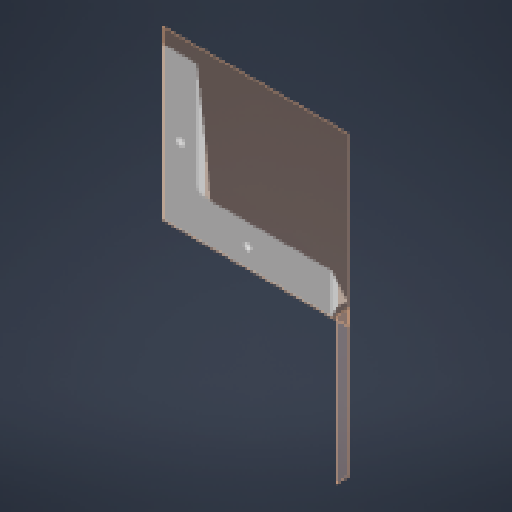
# Autodesk Inventor part: Base Gripper Support
Saved by Autodesk Inventor 2026.1 (Build 301233000, 233)
## iProperties
Created: 2025-11-01
Part Number: Base Gripper Support
Material: Generic
Document SubType Name: Modeling
Designer: rhema
Density: 1 g/cm^3
Appearance: Default
Mass: 7.12369 g
Surface Area: 52.7809 cm^2
Volume: 7.12369 cm^3
Author: rhema
Autodesk Inventor part; units mm, degrees
ref_plane "YZ Plane" through (0, 0, 0) normal (1, 0, 0) x (0, 1, 0)
ref_plane "XZ Plane" through (0, 0, 0) normal (0, 1, 0) x (-1, 0, 0)
ref_plane "XY Plane" through (0, 0, 0) normal (0, 0, 1) x (1, 0, 0)
ref_plane "Work Plane3" through (42.3, -5.3, -4.5) normal (1, 0, 0) x (0, 1, 0)
sketch "Sketch3" plane through (42.3, -5.3, -4.5) normal (1, 0, 0) x (0, 1, 0)
  line L0 (3.5, 2.5) -> (6, 0) projected
  line L1 (6, -5) -> (6, 0) projected
  line L2 (3.5, 2.5) -> (21.8, 2.5)
  line L3 (6, -5) -> (21.8, -5)
  line L4 (21.8, -5) -> (21.8, 2.5)
  line L5 (21.7, 2.4) -> (21.7, -4.9)
  line L6 (21.7, -4.9) -> (6.1, -4.9)
  line L7 (6.1, -4.9) -> (6.1, 0.0414)
  line L8 (6.1, 0.0414) -> (3.7414, 2.4)
  line L9 (3.7414, 2.4) -> (21.7, 2.4)
  point P0 (21.7, 2.4)
  dimension "d0" = 0.1
  dimension "d36" = 15.8
  dimension "d37" = 7.3
  dimension "d38" = 15.7
  dimension "d39" = 15.7
  dimension "d40" = 12.7986
  constraints: 16 end point, 3 perpendicular, 2 horizontal, 2 other
  measures "d0" distance between parallel lines of L3 L6
  measures "d36" distance between parallel lines of L1 L4
  measures "d37" distance of L5.start L5.end
  measures "d38" distance between parallel lines of L1 L5
  measures "d39" distance from line of point (21.7, 2.4) L1
  measures "d40" distance from line of point (21.7, 2.4) L0
extrude "Extrusion1" add sketch "Sketch3" against normal blind 75 contours L5 L6 L7 L8 L9
sketch "Sketch4" plane through (42.3, 16.4, -2.1) normal (0, 1, 0) x (1, 0, 0)
  line L0 (-60, -0.1) -> (-75, -0.1) projected
  line L1 (-75, -0.1) -> (-75, -7.1) projected
  line L2 (-60, 0) -> (-75, 0)
  line L3 (-75, 7.3) -> (-60, 7.3)
  arc A0 (-75, -7.1) -> (-70, -12.1) centre (-70, -7.1) ccw projected
  line L4 (-60, -12.1) -> (-70, -12.1) projected
  line L5 (-60, -0.1) -> (-60, -8.7171) projected
  line L6 (-60, -10.4829) -> (-60, -12.1) projected
  line L7 (-60, -10.4829) -> (-63.5, -11.1) projected
  line L8 (-63.5, -11.1) -> (-63.5, -8.1) projected
  line L9 (-63.5, -8.1) -> (-60, -8.7171) projected
  line L10 (-60, 0) -> (-60, 7.3)
  line L11 (-75, 0) -> (-75, 7.3)
  dimension "d41" = 15
  constraints: 8 end point, 1 horizontal, 1 parallel, 1 vertical
  measures "d41" distance between parallel lines of L11 L10
extrude "Extrusion2" add sketch "Sketch4" along normal blind 50 contours L2 L11 L3 L10
sketch "Sketch5" plane through (-32.7, -5.3, -4.5) normal (-1, 0, 0) x (0, 0, 1)
  line L0 (2.4, 3.7414) -> (2.4, 71.7) projected
  line L1 (2.4, 71.7) -> (2.4, 3.7414)
  line L2 (-4.9, 6.1) -> (0.0414, 6.1) projected
  line L3 (2.4, 3.7414) -> (0.0414, 6.1)
  line L4 (0.0414, 6.1) -> (-4.9, 6.1)
  line L5 (2.4, 71.7) -> (-4.9, 6.1)
  line L6 (2.4, 71.7) -> (-4.9, 71.7)
  line L7 (-4.9, 71.7) -> (-4.9, 6.1)
  constraints: 12 end point, 1 collinear, 1 horizontal, 1 perpendicular, 1 vertical
extrude "Extrusion3" cut sketch "Sketch5" against normal through all contours L5 L7 L6
sketch "Sketch6" plane through (42.3, -5.3, -4.5) normal (1, 0, 0) x (0, 0, -1)
  line L0 (3.164, 21.7) -> (-2.4, 71.7) projected
  line L1 (4.9, 6.1) -> (3.164, 21.7)
  line L2 (3.164, 21.7) -> (-2.4, 21.7)
  line L3 (-2.4, 3.7414) -> (-2.4, 71.7) projected
  line L4 (4.9, 6.1) -> (-2.4, 21.7)
  constraints: 6 end point, 1 collinear, 1 horizontal, 1 point on line
extrude "Extrusion4" cut sketch "Sketch6" against normal blind 60 contours L1 L4 L2
sketch "Sketch7" plane through (-32.7, -1.5586, -2.1) normal (0, 0, 1) x (1, 0, 0)
  line L0 (75, 0) -> (0, 0) projected
  line L1 (0, 0) -> (0, 67.9586) projected
  line L2 (0, 67.9586) -> (15, 67.9586) projected
  line L3 (15, 17.9586) -> (15, 67.9586) projected
  point P0 (32.7, 1.5586)
  point P1 (37.5, 8.5)
  point P2 (7.5, 33.9793)
  point P3 (15, 22.6774)
  dimension "d10" = 37.5
  dimension "d11" = 8.5
  dimension "d12" = 7.5
  dimension "d13" = 33.9793
  measures "d10" distance from line of L1 point (37.5, 8.5)
  measures "d11" distance from line of L0 point (37.5, 8.5)
  measures "d12" distance from line of L3 point (7.5, 33.979)
  measures "d13" distance from line of point (7.5, 33.979) L0
hole "Hole1" at (4.8, 6.9414, -2.1) at (-25.2, 32.4207, -2.1) direction (0, 0, -1) diameter 3.4 end through all clearance for "Flat Head Machine Screw" size "M3" standard "Ansi Metric M Profile"
ref_plane "Work Plane4" through (-32.7, -1.5586, -5.35) normal (0, 0, 1) x (1, 0, 0)
sketch "Sketch10" plane through (-32.7, -1.5586, -5.35) normal (0, 0, 1) x (1, 0, 0)
  point P0 (32.7, 1.5586)
  point P1 (37.5, 8.5)
  point P2 (7.5, 33.9793)
hole "Hole2" at (4.8, 6.9414, -5.35) at (-25.2, 32.4207, -5.35) direction (0, 0, -1) diameter 6 end through all
fillet "Fillet2" radius 2 1 edges at (-17.7, 8.6, -5.75)
body "Solid1"
